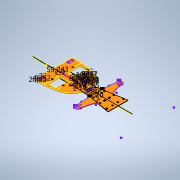
# Autodesk Inventor part: head_1
Saved by Autodesk Inventor 2020 (Build 240168000, 168)
## iProperties
Created: 2022-02-10
Part Number: head_1
Material: Типовые
Document SubType Name: Modeling
Designer: HP
Density: 1 g/cm^3
Appearance: Оранжевый
Mass: 318.083 g
Surface Area: 1630.63 cm^2
Volume: 318.083 cm^3
Author: HP
Autodesk Inventor part; units mm, degrees
ref_plane "YZ Plane" through (0, 0, 0) normal (1, 0, 0) x (0, 1, 0)
ref_plane "XZ Plane" through (0, 0, 0) normal (0, 1, 0) x (-1, 0, 0)
ref_plane "XY Plane" through (0, 0, 0) normal (0, 0, 1) x (1, 0, 0)
sketch "Эскиз1" plane through (0, 0, 0) normal (0, 1, 0) x (-1, 0, 0)
  line L0 (0, 0) -> (-339.521623, 0)
  line L1 (-129.027257, 2.001671) -> (-133.027257, 2.001671) construction
  line L2 (-133.027257, 20.919701) -> (-133.027257, 2.001671) construction
  line L3 (-133.027257, 20.919701) -> (-129.027257, 20.919701) construction
  line L4 (-129.027257, 20.919701) -> (-129.027257, 2.001671) construction
  line L5 (-129.027257, 2.001671) -> (-129.027257, -5.979416)
  line L6 (-10.109935, 0) -> (-40.109935, 0)
  line L7 (-53.743546, -154.136162) -> (-65.871746, -156.19724) construction
  line L8 (-65.871746, -156.19724) -> (-85.372712, -156.989963) construction
  line L9 (-85.372712, -156.989963) -> (-121.679389, -156.038696) construction
  line L10 (-121.679389, -156.038696) -> (-146.412322, -154.136162) construction
  line L11 (-146.412322, -154.136162) -> (-185.097168, -149.221285) construction
  line L12 (-185.097168, -149.221285) -> (-220.928211, -142.879507) construction
  line L13 (-220.928211, -142.879507) -> (-240.429178, -137.64754) construction
  line L14 (-240.429178, -137.64754) -> (-274.35769, -124.963985) construction
  line L15 (-274.35769, -124.963985) -> (-292.748845, -114.024418) construction
  line L16 (-292.748845, -114.024418) -> (-307.334934, -99.596873) construction
  line L17 (-307.334934, -99.596873) -> (-319.384311, -84.53515) construction
  line L18 (-319.384311, -84.53515) -> (-329.372611, -68.205072) construction
  line L19 (-329.372611, -68.205072) -> (-336.665655, -52.667716) construction
  line L20 (-336.665655, -52.667716) -> (-338.102036, -47.843891) construction
  spline S0 degree 4 poles (-53.743546, -154.136162) (-65.871746, -156.19724) (-85.372712, -156.989963) (-121.679389, -156.038696) (-146.412322, -154.136162) (-185.097168, -149.221285) (-220.928211, -142.879507) (-240.429178, -137.64754) (-274.35769, -124.963985) (-292.748845, -114.024418) (-307.334934, -99.596873) (-319.384311, -84.53515) (-329.372611, -68.205072) (-336.665655, -52.667716) (-338.102036, -47.843891) knots 1 1 1 1 1 2 3 4 5 6 7 8 9 10 11 12 12 12 12 12
  line L21 (-338.102036, -47.843891) -> (-338.102036, 0)
  line L22 (-53.743546, 154.136162) -> (-65.871746, 156.19724) construction
  line L23 (-65.871746, 156.19724) -> (-85.372712, 156.989963) construction
  line L24 (-85.372712, 156.989963) -> (-121.679389, 156.038696) construction
  line L25 (-121.679389, 156.038696) -> (-146.412322, 154.136162) construction
  line L26 (-146.412322, 154.136162) -> (-185.097168, 149.221285) construction
  line L27 (-185.097168, 149.221285) -> (-220.928211, 142.879507) construction
  line L28 (-220.928211, 142.879507) -> (-240.429178, 137.64754) construction
  line L29 (-240.429178, 137.64754) -> (-274.35769, 124.963985) construction
  line L30 (-274.35769, 124.963985) -> (-292.748845, 114.024418) construction
  line L31 (-292.748845, 114.024418) -> (-307.334934, 99.596873) construction
  line L32 (-307.334934, 99.596873) -> (-319.384311, 84.53515) construction
  line L33 (-319.384311, 84.53515) -> (-329.372611, 68.205072) construction
  line L34 (-329.372611, 68.205072) -> (-336.665655, 52.667716) construction
  line L35 (-336.665655, 52.667716) -> (-338.102036, 47.843891) construction
  spline S1 degree 4 poles (-53.743546, 154.136162) (-65.871746, 156.19724) (-85.372712, 156.989963) (-121.679389, 156.038696) (-146.412322, 154.136162) (-185.097168, 149.221285) (-220.928211, 142.879507) (-240.429178, 137.64754) (-274.35769, 124.963985) (-292.748845, 114.024418) (-307.334934, 99.596873) (-319.384311, 84.53515) (-329.372611, 68.205072) (-336.665655, 52.667716) (-338.102036, 47.843891) knots 1 1 1 1 1 2 3 4 5 6 7 8 9 10 11 12 12 12 12 12
  line L36 (-338.102036, 47.843891) -> (-338.102036, 0)
  line L37 (-144.743546, 0) -> (-53.743546, 0)
  line L38 (-53.743546, 0) -> (-53.743546, -154.136162)
  line L39 (-53.743546, 154.136162) -> (-65.871746, 156.19724) construction
  line L40 (-65.871746, 156.19724) -> (-85.372712, 156.989963) construction
  line L41 (-85.372712, 156.989963) -> (-121.679389, 156.038696) construction
  line L42 (-121.679389, 156.038696) -> (-146.412322, 154.136162) construction
  line L43 (-146.412322, 154.136162) -> (-185.097168, 149.221285) construction
  line L44 (-185.097168, 149.221285) -> (-220.928211, 142.879507) construction
  line L45 (-220.928211, 142.879507) -> (-240.429178, 137.64754) construction
  line L46 (-240.429178, 137.64754) -> (-274.35769, 124.963985) construction
  line L47 (-274.35769, 124.963985) -> (-292.748845, 114.024418) construction
  line L48 (-292.748845, 114.024418) -> (-307.334934, 99.596873) construction
  line L49 (-307.334934, 99.596873) -> (-319.384311, 84.53515) construction
  line L50 (-319.384311, 84.53515) -> (-329.372611, 68.205072) construction
  line L51 (-329.372611, 68.205072) -> (-336.665655, 52.667716) construction
  line L52 (-336.665655, 52.667716) -> (-338.102036, 47.843891) construction
  spline S2 degree 4 poles (-53.743546, 154.136162) (-65.871746, 156.19724) (-85.372712, 156.989963) (-121.679389, 156.038696) (-146.412322, 154.136162) (-185.097168, 149.221285) (-220.928211, 142.879507) (-240.429178, 137.64754) (-274.35769, 124.963985) (-292.748845, 114.024418) (-307.334934, 99.596873) (-319.384311, 84.53515) (-329.372611, 68.205072) (-336.665655, 52.667716) (-338.102036, 47.843891) knots 1 1 1 1 1 2 3 4 5 6 7 8 9 10 11 12 12 12 12 12
  line L53 (-338.102036, 47.843891) -> (-338.102036, 0)
  line L54 (-53.743546, 0) -> (-53.743546, 154.136162)
  point P0 (-144.743546, 57.777799)
  dimension "d42" = 30
  constraints: 18 end point, 15 symmetric about line, 5 point on line, 2 perpendicular, 1 horizontal, 1 vertical, 9 other
  measures "d42" distance of L6.start L6.end
extrude "Выдавливание1" add sketch "Эскиз1" along normal blind 6
sketch "Эскиз2" plane through (0, 0, 0) normal (0, -1, 0) x (1, 0, 0)
  line L0 (218.921453, 99.86161) -> (218.921453, 139.806254)
  line L1 (218.921453, 139.806254) -> (222.921453, 139.806254)
  line L2 (222.921453, 139.806254) -> (222.921453, 99.86161)
  line L3 (218.921453, 99.86161) -> (222.921453, 99.86161)
  line L4 (218.921453, 59.916966) -> (222.921453, 59.916966)
  line L5 (218.921453, 19.972322) -> (218.921453, 59.916966)
  line L6 (222.921453, 59.916966) -> (222.921453, 19.972322)
  line L7 (218.921453, 19.972322) -> (222.921453, 19.972322)
  line L8 (218.921453, 84.547313) -> (218.921453, 87.447313) construction
  line L9 (222.921453, 87.447313) -> (222.921453, 84.547313) construction
  line L10 (0, 0) -> (287.43499, 0) construction
  line L11 (218.921453, 84.547313) -> (222.921453, 84.547313) construction
  line L12 (222.921453, 84.547313) -> (222.921453, 87.447313) construction
  line L13 (222.921453, 87.447313) -> (218.921453, 87.447313) construction
  line L14 (218.921453, 87.447313) -> (218.921453, 84.547313) construction
  line L15 (218.921453, 84.547313) -> (222.921453, 87.447313) construction
  line L16 (222.921453, 84.547313) -> (218.921453, 87.447313) construction
  circle A0 centre (220.921453, 85.997313) radius 1.5
  line L17 (218.921453, -99.86161) -> (218.921453, -139.806254)
  line L18 (218.921453, -139.806254) -> (222.921453, -139.806254)
  line L19 (222.921453, -139.806254) -> (222.921453, -99.86161)
  line L20 (218.921453, -99.86161) -> (222.921453, -99.86161)
  line L21 (218.921453, -59.916966) -> (222.921453, -59.916966)
  line L22 (218.921453, -19.972322) -> (218.921453, -59.916966)
  line L23 (222.921453, -59.916966) -> (222.921453, -19.972322)
  line L24 (218.921453, -19.972322) -> (222.921453, -19.972322)
  line L25 (218.921453, -84.547313) -> (218.921453, -87.447313) construction
  line L26 (222.921453, -87.447313) -> (222.921453, -84.547313) construction
  line L27 (218.921453, -84.547313) -> (222.921453, -84.547313) construction
  line L28 (222.921453, -84.547313) -> (222.921453, -87.447313) construction
  line L29 (222.921453, -87.447313) -> (218.921453, -87.447313) construction
  line L30 (218.921453, -87.447313) -> (218.921453, -84.547313) construction
  line L31 (218.921453, -84.547313) -> (222.921453, -87.447313) construction
  line L32 (222.921453, -84.547313) -> (218.921453, -87.447313) construction
  circle A1 centre (220.921453, -85.997313) radius 1.5
  dimension "d101" = 3
  constraints: 66 end point, 16 symmetric about line, 6 horizontal, 6 vertical, 4 midpoint, 2 centre point, 2 coincident, 2 parallel, 1 perpendicular, 13 other
  measures "d101" diameter of A0
sketch "Эскиз6" plane through (0, 0, 0) normal (0, -1, 0) x (1, 0, 0)
  line L0 (74.395998, 0) -> (255.779052, 0)
  line L1 (174.802002, 33.285159) -> (169.607709, 33.285159)
  line L2 (180.665084, 129.150848) -> (169.607709, 129.150848)
  line L3 (145.357709, 104.101025) -> (145.357709, 81.101025)
  line L4 (142.506422, 31.26111) -> (204.162039, 31.26111)
  line L5 (204.162039, 31.26111) -> (204.162039, 131.44265)
  line L6 (204.162039, 131.44265) -> (142.506422, 131.44265)
  line L7 (142.506422, 131.44265) -> (142.506422, 31.26111)
  line L8 (174.802002, -33.285159) -> (169.607709, -33.285159)
  line L9 (180.665084, -129.150848) -> (169.607709, -129.150848)
  line L10 (145.357709, -104.101025) -> (145.357709, -81.101025)
  line L11 (142.506422, -31.26111) -> (204.162039, -31.26111)
  line L12 (204.162039, -31.26111) -> (204.162039, -131.44265)
  line L13 (204.162039, -131.44265) -> (142.506422, -131.44265)
  line L14 (142.506422, -131.44265) -> (142.506422, -31.26111)
  point P0 (0, 0)
  constraints: 24 end point, 10 symmetric about line, 2 horizontal, 2 parallel, 1 perpendicular
sketch "Эскиз7" plane through (0, 0, 0) normal (0, -1, 0) x (1, 0, 0)
  point P0 (0, 0)
extrude "Выдавливание10" cut sketch "Эскиз6" against normal through all
sketch "Эскиз11" plane through (0, 6, 0) normal (0, 1, 0) x (1, 0, 0)
  line L0 (53.743546, 154.136162) -> (53.743546, -154.136162)
  line L1 (338.102036, -47.843891) -> (338.102036, 47.843891)
  point P0 (0, 0)
  constraints: 2 other
sketch "Эскиз12" plane through (0, 0, 0) normal (0, -1, 0) x (1, 0, 0)
  line L0 (232.5, 139.475161) -> (232.5, 54.475161)
  circle A0 centre (232.5, 54.475161) radius 0.05
  point P0 (0, 0)
  dimension "d56" = 85
  dimension "d60" = 0.1
  constraints: 2 coincident, 2 end point, 1 centre point, 1 vertical, 2 other
  measures "d56" distance of L0.start L0.end
  measures "d60" diameter of A0
extrude "Выдавливание12" cut sketch "Эскиз12" against normal blind 0.1
sketch "Эскиз13" plane through (0, 6, 0) normal (0, 1, 0) x (1, 0, 0)
  point P0 (0, 0)
  point P1 (303.305898, -69.722631)
sketch "Эскиз18" plane through (0, 0, 0) normal (0, -1, 0) x (1, 0, 0)
  line L0 (127.94871, -106.917014) -> (127.94871, -149.683819)
  line L1 (131.94871, -149.683819) -> (131.94871, -106.917014)
  line L2 (127.94871, -149.683819) -> (131.94871, -149.683819)
  line L3 (131.94871, -106.917014) -> (127.94871, -106.917014)
  line L4 (127.94871, -64.150208) -> (131.94871, -64.150208)
  line L5 (127.94871, -21.383403) -> (127.94871, -64.150208)
  line L6 (131.94871, -64.150208) -> (131.94871, -21.383403)
  line L7 (131.94871, -21.383403) -> (127.94871, -21.383403)
  line L8 (127.94871, -86.983611) -> (127.94871, -84.083611) construction
  line L9 (131.94871, -84.083611) -> (131.94871, -86.983611) construction
  line L10 (127.94871, -86.983611) -> (131.94871, -86.983611) construction
  line L11 (131.94871, -86.983611) -> (131.94871, -84.083611) construction
  line L12 (131.94871, -84.083611) -> (127.94871, -84.083611) construction
  line L13 (127.94871, -84.083611) -> (127.94871, -86.983611) construction
  line L14 (127.94871, -86.983611) -> (131.94871, -84.083611) construction
  line L15 (131.94871, -86.983611) -> (127.94871, -84.083611) construction
  circle A0 centre (129.94871, -85.533611) radius 1.5
  line L16 (0, 0) -> (309.38051, 0) construction
  line L17 (127.94871, 106.917014) -> (127.94871, 149.683819)
  line L18 (131.94871, 149.683819) -> (131.94871, 106.917014)
  line L19 (127.94871, 149.683819) -> (131.94871, 149.683819)
  line L20 (131.94871, 106.917014) -> (127.94871, 106.917014)
  line L21 (127.94871, 64.150208) -> (131.94871, 64.150208)
  line L22 (127.94871, 21.383403) -> (127.94871, 64.150208)
  line L23 (131.94871, 64.150208) -> (131.94871, 21.383403)
  line L24 (131.94871, 21.383403) -> (127.94871, 21.383403)
  line L25 (127.94871, 86.983611) -> (127.94871, 84.083611) construction
  line L26 (131.94871, 84.083611) -> (131.94871, 86.983611) construction
  line L27 (127.94871, 86.983611) -> (131.94871, 86.983611) construction
  line L28 (131.94871, 86.983611) -> (131.94871, 84.083611) construction
  line L29 (131.94871, 84.083611) -> (127.94871, 84.083611) construction
  line L30 (127.94871, 84.083611) -> (127.94871, 86.983611) construction
  line L31 (127.94871, 86.983611) -> (131.94871, 84.083611) construction
  line L32 (131.94871, 86.983611) -> (127.94871, 84.083611) construction
  circle A1 centre (129.94871, 85.533611) radius 1.5
  dimension "d96" = 3
  constraints: 66 end point, 16 symmetric about line, 6 horizontal, 6 vertical, 4 midpoint, 2 centre point, 2 coincident, 2 parallel, 1 perpendicular, 13 other
  measures "d96" diameter of A0
extrude "Выдавливание22" cut sketch "Эскиз18" against normal blind 10
extrude "Выдавливание23" cut sketch "Эскиз2" against normal through all
sketch "Эскиз19" plane through (0, 6, 0) normal (0, 1, 0) x (1, 0, 0)
  line L0 (590.53404, -82.183099) -> (370.53404, -45)
  line L1 (590.53404, 82.183099) -> (590.53404, -82.183099) construction
  line L2 (370.53404, -45) -> (204.162039, -45)
  line L3 (590.53404, 0) -> (590.53404, -82.183099)
  line L4 (222.921453, 139.806254) -> (222.921453, 99.86161)
  line L5 (222.921453, 99.86161) -> (218.921453, 99.86161)
  line L6 (218.921453, 99.86161) -> (218.921453, 139.806254)
  line L7 (218.921453, 139.806254) -> (222.921453, 139.806254)
  circle A0 centre (220.921453, -85.997313) radius 1.5
  line L8 (222.921453, -139.806254) -> (218.921453, -139.806254)
  line L9 (218.921453, -139.806254) -> (218.921453, -99.86161)
  line L10 (218.921453, -99.86161) -> (222.921453, -99.86161)
  line L11 (222.921453, -99.86161) -> (222.921453, -139.806254)
  line L12 (222.921453, 19.972322) -> (218.921453, 19.972322)
  line L13 (218.921453, 19.972322) -> (218.921453, 59.916966)
  line L14 (218.921453, 59.916966) -> (222.921453, 59.916966)
  line L15 (222.921453, 59.916966) -> (222.921453, 19.972322)
  circle A1 centre (220.921453, 85.997313) radius 1.5
  line L16 (218.921453, -19.972322) -> (222.921453, -19.972322)
  line L17 (222.921453, -19.972322) -> (222.921453, -59.916966)
  line L18 (222.921453, -59.916966) -> (218.921453, -59.916966)
  line L19 (218.921453, -59.916966) -> (218.921453, -19.972322)
  line L20 (127.94871, 106.917014) -> (127.94871, 149.683819)
  line L21 (127.94871, 149.683819) -> (131.94871, 149.683819)
  line L22 (131.94871, 149.683819) -> (131.94871, 106.917014)
  line L23 (131.94871, 106.917014) -> (127.94871, 106.917014)
  line L24 (127.94871, -21.383403) -> (131.94871, -21.383403)
  line L25 (131.94871, -21.383403) -> (131.94871, -64.150208)
  line L26 (131.94871, -64.150208) -> (127.94871, -64.150208)
  line L27 (127.94871, -64.150208) -> (127.94871, -21.383403)
  line L28 (127.94871, 21.383403) -> (127.94871, 64.150208)
  line L29 (127.94871, 64.150208) -> (131.94871, 64.150208)
  line L30 (131.94871, 64.150208) -> (131.94871, 21.383403)
  line L31 (131.94871, 21.383403) -> (127.94871, 21.383403)
  circle A2 centre (129.94871, 85.533611) radius 1.5
  circle A3 centre (129.94871, -85.533611) radius 1.5
  line L32 (127.94871, -149.683819) -> (127.94871, -106.917014)
  line L33 (127.94871, -106.917014) -> (131.94871, -106.917014)
  line L34 (131.94871, -106.917014) -> (131.94871, -149.683819)
  line L35 (131.94871, -149.683819) -> (127.94871, -149.683819)
  line L36 (132.908073, -2) -> (132.908073, 2)
  line L37 (132.908073, 2) -> (192.597533, 2)
  line L38 (192.597533, 2) -> (192.597533, -2)
  line L39 (192.597533, -2) -> (132.908073, -2)
  circle A4 centre (252.499965, -54.504877) radius 1.5
  circle A5 centre (252.489072, -26.566338) radius 1.5
  circle A6 centre (304.82708, -21.46988) radius 1.5
  line L40 (204.162039, -31.26111) -> (204.162039, -131.44265)
  line L41 (204.162039, -131.44265) -> (142.506422, -131.44265)
  line L42 (142.506422, -131.44265) -> (142.506422, -31.26111)
  line L43 (142.506422, -31.26111) -> (204.162039, -31.26111)
  line L44 (204.162039, 31.26111) -> (142.506422, 31.26111)
  line L45 (142.506422, 31.26111) -> (142.506422, 131.44265)
  line L46 (142.506422, 131.44265) -> (204.162039, 131.44265)
  line L47 (204.162039, 131.44265) -> (204.162039, 31.26111)
  line L48 (338.102036, -47.843891) -> (338.102036, 47.843891)
  spline S0 degree 4 poles (338.102036, 47.843891) (336.665655, 52.667716) (329.372611, 68.205072) (319.384311, 84.53515) (307.334934, 99.596873) (292.748845, 114.024418) (274.35769, 124.963985) (240.429178, 137.64754) (220.928211, 142.879507) (185.097168, 149.221285) (146.412322, 154.136162) (121.679389, 156.038696) (85.372712, 156.989963) (65.871746, 156.19724) (53.743546, 154.136162) knots 1 1 1 1 1 2 3 4 5 6 7 8 9 10 11 12 12 12 12 12
  line L49 (53.743546, 154.136162) -> (53.743546, -154.136162)
  spline S1 degree 4 poles (53.743546, -154.136162) (65.871746, -156.19724) (85.372712, -156.989963) (121.679389, -156.038696) (146.412322, -154.136162) (185.097168, -149.221285) (220.928211, -142.879507) (240.429178, -137.64754) (274.35769, -124.963985) (292.748845, -114.024418) (307.334934, -99.596873) (319.384311, -84.53515) (329.372611, -68.205072) (336.665655, -52.667716) (338.102036, -47.843891) knots 1 1 1 1 1 2 3 4 5 6 7 8 9 10 11 12 12 12 12 12
  circle A7 centre (366.494375, -34.175417) radius 1.5
  circle A8 centre (433.543463, -45.507657) radius 1.5
  circle A9 centre (433.543463, -22.843176) radius 1.5
  circle A10 centre (500.592552, -56.839897) radius 1.5
  circle A11 centre (500.592552, -22.843176) radius 1.5
  circle A12 centre (500.592552, -14.75) radius 1.45
  circle A13 centre (567.641641, -68.172138) radius 1.5
  circle A14 centre (567.641641, -22.843176) radius 1.5
  circle A15 centre (366.494375, 0) radius 1.5
  line L50 (590.53404, 0) -> (556.709794, 0)
  line L51 (590.53404, 0) -> (557.964133, 0)
  line L52 (590.53404, 82.183099) -> (370.53404, 45)
  line L53 (590.53404, 0) -> (590.53404, 82.183099)
  circle A16 centre (366.494375, 34.175417) radius 1.5
  circle A17 centre (433.543463, 45.507657) radius 1.5
  circle A18 centre (433.543463, 22.843176) radius 1.5
  circle A19 centre (500.592552, 56.839897) radius 1.5
  circle A20 centre (500.592552, 22.843176) radius 1.5
  circle A21 centre (500.592552, 14.75) radius 1.45
  circle A22 centre (567.641641, 68.172138) radius 1.5
  circle A23 centre (567.641641, 22.843176) radius 1.5
  circle A24 centre (366.494375, 0) radius 1.5
  line L54 (370.53404, 45) -> (204.162039, 45)
  line L55 (204.162039, -31.26111) -> (204.162039, -131.44265)
  line L56 (204.162039, 131.44265) -> (204.162039, 31.26111)
  circle A25 centre (348.506066, -17.087708) radius 8
  circle A26 centre (304.839956, -21.484903) radius 1.5
  circle A27 centre (303.29996, -69.744885) radius 1.5
  circle A28 centre (252.499965, -26.564858) radius 1.5
  circle A29 centre (252.499965, -54.504877) radius 1.5
  line L57 (366.494375, -34.175417) -> (366.494375, 0)
  line L58 (-118.106808, 0) -> (708.640848, 0)
  circle A30 centre (348.506066, 17.087708) radius 8
  circle A31 centre (348.506066, -17.087708) radius 9.5
  circle A32 centre (348.506066, 17.087708) radius 9.5
  line L59 (366.494375, -34.175417) -> (434.494375, -34.175417) construction
  circle A33 centre (299.444666, -22.846844) radius 1.5
  line L60 (299.444666, -22.846844) -> (367.444666, -22.846844) construction
  circle A34 centre (232.394957, -11.518271) radius 1.5
  circle A35 centre (299.444666, 22.846844) radius 1.5
  circle A36 centre (232.394957, 11.518271) radius 1.5
  point P0 (0, 0)
  point P1 (338.102036, 45)
  point P2 (338.102036, -45)
  point P3 (305.972405, -20.501257)
  point P4 (303.694631, -22.453526)
  point P5 (252.292545, -25.079268)
  point P6 (252.696492, -28.051928)
  point P7 (366.494375, -17.087708)
  dimension "d118" = 16
  dimension "d190" = 19
  dimension "d215" = 3
  constraints: 37 centre point, 24 end point, 12 symmetric about line, 5 equal radius, 5 horizontal, 3 vertical, 2 coincident, 2 midpoint, 1 point on line, 39 other
  measures "d118" diameter of A25
  measures "d190" diameter of A31
  measures "d215" diameter of A33
sketch "Эскиз20" plane through (0, 6, 0) normal (0, 1, 0) x (1, 0, 0)
  line L0 (338.102036, -47.843891) -> (338.102036, 47.843891)
  line L1 (370.53404, -45) -> (150.53404, -45)
  line L2 (338.102036, -45) -> (398.310009, -45) construction
  circle A0 centre (313.494375, 0) radius 1.5
  circle A1 centre (313.494375, 0) radius 1.5
  line L3 (313.494375, 0) -> (378.494375, 0)
  circle A2 centre (378.494375, 0) radius 2.5
  line L4 (378.494375, 0) -> (408.494375, 0)
  line L5 (590.53404, -82.183099) -> (496.225076, -66.243556)
  line L6 (370.53404, 45) -> (590.53404, 82.183099)
  line L7 (150.53404, 45) -> (370.53404, 45)
  line L8 (408.494375, 0) -> (408.494375, -51.415831)
  line L9 (408.494375, 51.415831) -> (408.494375, 0)
  spline S0 degree 2 poles (408.494375, -51.415831) (407.497612, -115.458679) (417.984162, -180.733061) knots 0 0 0 1 1 1
  arc A3 (417.984162, -180.733061) -> (450.061396, -183.259047) centre (434.721088, -173.128293) ccw
  spline S1 degree 2 poles (408.494375, 51.415831) (407.497612, 115.458679) (417.984162, 180.733061) knots 0 0 0 1 1 1
  arc A4 (450.061396, 183.259047) -> (417.984162, 180.733061) centre (434.721088, 173.128293) ccw
  line L10 (590.53404, -82.183099) -> (370.53404, -45)
  line L11 (338.102036, -47.843891) -> (338.102036, 47.843891)
  line L12 (313.494375, 0) -> (338.102036, 0)
  line L13 (708.640848, 0) -> (-118.106808, 0)
  line L14 (53.743546, 154.136162) -> (53.743546, -154.136162)
  line L15 (53.743546, 0) -> (112.615546, 0)
  line L16 (53.743546, 0) -> (112.986546, 0)
  line L17 (112.986546, 0) -> (110.086546, 0)
  circle A5 centre (111.536546, 0) radius 1.45
  line L18 (460.711317, -60.24123) -> (480.431637, -63.574242)
  arc A6 (474.217889, -78.803208) -> (450.061396, -183.259047) centre (835.740939, -217.43029) ccw
  arc A7 (496.225076, -66.243556) -> (474.217889, -78.803208) centre (492.892065, -85.963876) ccw
  arc A8 (450.061396, 183.259047) -> (417.984162, 180.733061) centre (434.721088, 173.128293) ccw
  arc A9 (450.061396, 183.259047) -> (474.217889, 78.803208) centre (835.740939, 217.43029) ccw
  arc A10 (474.217889, 78.803208) -> (496.225076, 66.243556) centre (492.892065, 85.963876) ccw
  point P0 (0, 0)
  point P1 (453.008626, -171.251285)
  point P2 (432.734599, -153.77409)
  point P3 (453.008626, 171.251285)
  point P4 (432.734599, 153.77409)
  point P5 (450.863733, 150.353763)
  dimension "d106" = 65
  dimension "d107" = 5
  dimension "d110" = 30
  dimension "d225" = 3
  dimension "d240" = 59.243
  dimension "d241" = 2.9
  dimension "d260" = 20
  constraints: 30 end point, 15 point on circle, 10 centre point, 9 point on line, 6 vertical alignment, 5 symmetric about line, 4 horizontal, 3 equal radius, 3 midpoint, 2 coincident, 2 tangent, 1 collinear, 1 horizontal alignment, 1 perpendicular, 1 vertical, 28 other
  measures "d106" distance of L3.start L3.end
  measures "d107" diameter of A2
  measures "d110" distance of L4.start L4.end
  measures "d225" diameter of A0
  measures "d240" distance of L15.start L16.end
  measures "d241" distance of L16.end L17.end
  measures "d260" radius of A7
extrude "Выдавливание24" add sketch "Эскиз19" against normal blind 6 contours L0 L2 L48 L58 A15 L50 L3 | L50 L58 A15 L48 L54 L52 L53 | A25 | A30 | A31 | A32
extrude "Выдавливание25" add sketch "Эскиз20" against normal blind 6 contours L10 A7 A6 A3 S0
sketch "Эскиз34" plane through (0, 0, 0) normal (0, -1, 0) x (1, 0, 0)
  line L0 (147.451162, 2) -> (147.451162, -2)
  line L1 (147.451162, -2) -> (194.844244, -2)
  line L2 (194.844244, 2) -> (147.451162, 2)
  line L3 (194.844244, -2) -> (194.844244, 2)
  line L4 (242.237326, 2) -> (242.237326, -2)
  line L5 (242.237326, -2) -> (289.630407, -2)
  line L6 (289.630407, 2) -> (242.237326, 2)
  line L7 (289.630407, -2) -> (289.630407, 2)
  line L8 (52.664999, -2) -> (100.058081, -2)
  line L9 (100.058081, 2) -> (52.664999, 2)
  line L10 (100.058081, -2) -> (100.058081, 2)
  line L11 (52.664999, 2) -> (52.664999, -2)
  point P0 (0, 0)
  constraints: 24 end point, 6 horizontal, 6 vertical, 12 other
extrude "Выдавливание43" cut sketch "Эскиз34" against normal blind 6
extrude "Выдавливание26" cut sketch "Эскиз20" against normal blind 6 contours A2 L4 L3 | L3 L4 A2 | L3 L13 A0 | A0 L13 L3
extrude "Выдавливание27" cut sketch "Эскиз19" against normal blind 6 contours A25
sketch "Эскиз21" plane through (0, 6, 0) normal (0, 1, 0) x (1, 0, 0)
  point P0 (0, 0)
sketch "Эскиз22" plane through (0, 6, 0) normal (0, 1, 0) x (1, 0, 0)
  line L0 (272.616718, 69.365757) -> (272.616718, 26.185757)
  line L1 (272.616718, 26.185757) -> (293.698718, 26.185757)
  line L2 (293.698718, 26.185757) -> (293.698718, 69.365757)
  line L3 (293.698718, 69.365757) -> (272.616718, 69.365757)
  line L4 (293.698718, 69.365757) -> (293.698718, 62.761757)
  line L5 (283.157718, 69.365757) -> (291.730218, 69.365757)
  circle A0 centre (291.730218, 62.761757) radius 1.44
  line L6 (272.616718, 26.185757) -> (272.616718, 32.789757)
  circle A1 centre (274.585303, 33.099696) radius 1.44
  line L7 (293.698718, 62.761757) -> (293.170218, 62.761757)
  line L8 (246.593604, 26.185757) -> (246.593604, 69.365757)
  line L9 (246.593604, 69.365757) -> (225.511604, 69.365757)
  line L10 (225.511604, 69.365757) -> (225.511604, 26.185757)
  line L11 (225.511604, 26.185757) -> (246.593604, 26.185757)
  line L12 (294.698803, 68.675696) -> (294.698803, 62.071696)
  line L13 (236.052604, 26.185757) -> (227.480104, 26.185757)
  circle A2 centre (227.480104, 32.789757) radius 1.44
  circle A3 centre (244.625104, 62.761757) radius 1.44
  line L14 (294.698803, 62.071696) -> (294.170303, 62.071696)
  circle A4 centre (251.765737, 32.789757) radius 1.44
  line L15 (249.816991, 26.185757) -> (270.898991, 26.185757)
  line L16 (249.816991, 69.365757) -> (249.816991, 26.185757)
  line L17 (270.898991, 26.185757) -> (270.898991, 69.365757)
  circle A5 centre (268.680505, 62.761757) radius 1.44
  line L18 (270.898991, 69.365757) -> (249.816991, 69.365757)
  line L19 (227.480104, 26.185757) -> (227.480104, 32.789757)
  line L20 (227.480104, 32.789757) -> (225.511604, 32.789757)
  line L21 (268.680505, 62.761757) -> (268.680505, 69.365757)
  line L22 (244.625104, 62.761757) -> (244.625104, 69.365757)
  line L23 (251.765737, 32.789757) -> (251.765737, 26.185757)
  line L24 (246.593604, 69.365757) -> (244.625104, 69.365757)
  point P0 (0, 0)
  point P1 (294.170303, 62.071696)
  point P2 (295.170303, 61.071696)
  dimension "d125" = 2.88
  dimension "d121" = 43.18
  dimension "d122" = 21.082
  dimension "d123" = 6.604
  dimension "d124" = 8.5725
  dimension "d126" = 6.604
  dimension "d128" = 2.88
  dimension "d129" = 0.5285
  dimension "d156" = 21.082
  dimension "d157" = 6.604
  dimension "d158" = 8.5725
  dimension "d159" = 2.88
  dimension "d163" = 0.5285
  dimension "d171" = 43.18
  dimension "d175" = 6.604
  dimension "d176" = 1.9685
  constraints: 50 end point, 11 parallel, 8 point on line, 6 perpendicular, 5 centre point, 3 equal radius, 2 collinear, 2 midpoint, 1 horizontal alignment, 2 other
  measures "d121" distance of L2.end L1.end
  measures "d122" distance of L1.end L0.end
  measures "d123" distance of L2.end L4.end
  measures "d124" distance of L5.start L5.end
  measures "d126" distance of L0.end L6.end
  measures "d128" diameter of A1
  measures "d129" distance of L4.end L7.end
  measures "d156" distance of L9.end L9.start
  measures "d157" distance of L12.start L14.start
  measures "d158" distance of L13.start L13.end
  measures "d159" diameter of A2
  measures "d163" distance of L14.start L14.end
  measures "d171" distance of L8.start L9.start
  measures "d175" distance of L22.start L22.end
  measures "d176" distance of L9.start L22.end
extrude "Выдавливание28" cut sketch "Эскиз22" against normal blind 6 contours A0 | A1
sketch "Эскиз19 outline for Выдавливание29" plane through (0, 6, 0) normal (0, 1, 0) x (1, 0, 0)
  arc A0 (305.972405, -20.501257) -> (303.694631, -22.453526) centre (304.839956, -21.484903) ccw
  arc A1 (303.694631, -22.453526) -> (305.972405, -20.501257) centre (304.82708, -21.46988) ccw
  arc A2 (252.292545, -25.079268) -> (252.696492, -28.051928) centre (252.499965, -26.564858) ccw
  arc A3 (252.696492, -28.051928) -> (252.292545, -25.079268) centre (252.489072, -26.566338) ccw
  circle A4 centre (303.29996, -69.744885) radius 1.5
  circle A5 centre (252.499965, -54.504877) radius 1.5
extrude "Выдавливание29" cut sketch "Эскиз19 outline for Выдавливание29" against normal blind 6
sketch "Эскиз24" plane through (0, 6, 0) normal (0, 1, 0) x (1, 0, 0)
  circle A0 centre (252.499965, -54.504877) radius 1.5
  circle A1 centre (252.489072, -26.566338) radius 1.5
  circle A2 centre (304.82708, -21.46988) radius 1.5
  circle A3 centre (304.839956, -21.484903) radius 1.5
  circle A4 centre (303.29996, -69.744885) radius 1.5
  circle A5 centre (252.499965, -26.564858) radius 1.5
  circle A6 centre (252.499965, -54.504877) radius 1.5
  circle A7 centre (252.499965, -54.504877) radius 1.5
  circle A8 centre (252.489072, -26.566338) radius 1.5
  circle A9 centre (304.82708, -21.46988) radius 1.5
  circle A10 centre (304.839956, -21.484903) radius 1.5
  circle A11 centre (303.29996, -69.744885) radius 1.5
  circle A12 centre (252.499965, -26.564858) radius 1.5
  circle A13 centre (252.499965, -54.504877) radius 1.5
  point P0 (0, 0)
  dimension "d141" = 3
  dimension "d142" = 3
  constraints: 20 centre point, 6 equal radius
  measures "d141" diameter of A3
  measures "d142" diameter of A10
sketch "Эскиз25" plane through (0, 6, 0) normal (0, 1, 0) x (1, 0, 0)
  circle A0 centre (81.981142, 102.339991) radius 1.5
  circle A1 centre (109.91968, 102.350884) radius 1.5
  circle A2 centre (115.016139, 50.012877) radius 1.5
  circle A3 centre (115.001115, 50) radius 1.5
  circle A4 centre (66.50538, 51.540412) radius 1.5
  circle A5 centre (109.92116, 102.339991) radius 1.5
  circle A6 centre (81.981142, 102.339991) radius 1.5
  line L0 (-118.106808, 0) -> (708.640848, 0)
  circle A7 centre (99.304624, -100.798453) radius 1.5
  circle A8 centre (115.001115, -50) radius 1.5
  circle A9 centre (66.50538, -48.471755) radius 1.5
  circle A10 centre (71.364605, -100.798453) radius 1.5
  line L1 (132.908073, -2) -> (132.908073, 2)
  line L2 (69.825662, -13.240842) -> (71.825662, -13.240842)
  line L3 (71.825662, -13.240842) -> (71.825662, -9.240842)
  line L4 (71.825662, -9.240842) -> (69.825662, -9.240842)
  line L5 (69.825662, -9.240842) -> (69.825662, -13.240842)
  line L6 (86.825662, -13.240842) -> (88.825662, -13.240842)
  line L7 (88.825662, -13.240842) -> (88.825662, -9.240842)
  line L8 (88.825662, -9.240842) -> (86.825662, -9.240842)
  line L9 (86.825662, -9.240842) -> (86.825662, -13.240842)
  line L10 (69.825662, 13.240842) -> (71.825662, 13.240842)
  line L11 (71.825662, 13.240842) -> (71.825662, 9.240842)
  line L12 (71.825662, 9.240842) -> (69.825662, 9.240842)
  line L13 (69.825662, 9.240842) -> (69.825662, 13.240842)
  line L14 (86.825662, 13.240842) -> (88.825662, 13.240842)
  line L15 (88.825662, 13.240842) -> (88.825662, 9.240842)
  line L16 (88.825662, 9.240842) -> (86.825662, 9.240842)
  line L17 (86.825662, 9.240842) -> (86.825662, 13.240842)
  line L18 (251.413455, 11.187786) -> (253.413455, 11.187786)
  line L19 (253.413455, 11.187786) -> (253.413455, 15.187786)
  line L20 (253.413455, 15.187786) -> (251.413455, 15.187786)
  line L21 (251.413455, 15.187786) -> (251.413455, 11.187786)
  line L22 (268.413455, 11.187786) -> (270.413455, 11.187786)
  line L23 (270.413455, 11.187786) -> (270.413455, 15.187786)
  line L24 (270.413455, 15.187786) -> (268.413455, 15.187786)
  line L25 (268.413455, 15.187786) -> (268.413455, 11.187786)
  line L26 (117.431454, 26.92188) -> (97.431454, 26.92188)
  line L27 (97.431454, 26.92188) -> (97.431454, 6.92188)
  line L28 (97.431454, 6.92188) -> (117.431454, 6.92188)
  line L29 (117.431454, 6.92188) -> (117.431454, 26.92188)
  line L30 (97.431454, 16.92188) -> (99.435231, 16.92188)
  line L31 (99.435231, 16.92188) -> (99.435231, 7.62188)
  line L32 (99.435231, 7.62188) -> (99.435231, 26.22188)
  circle A11 centre (99.435231, 7.62188) radius 0.5
  circle A12 centre (99.435231, 26.22188) radius 0.5
  line L33 (117.431454, -26.92188) -> (97.431454, -26.92188)
  line L34 (97.431454, -26.92188) -> (97.431454, -6.92188)
  line L35 (97.431454, -6.92188) -> (117.431454, -6.92188)
  line L36 (117.431454, -6.92188) -> (117.431454, -26.92188)
  line L37 (97.431454, -16.92188) -> (99.435231, -16.92188)
  line L38 (99.435231, -16.92188) -> (99.435231, -7.62188)
  line L39 (99.435231, -7.62188) -> (99.435231, -26.22188)
  circle A13 centre (99.435231, -7.62188) radius 0.5
  circle A14 centre (99.435231, -26.22188) radius 0.5
  point P0 (0, 0)
  point P1 (111.40675, 102.547411)
  point P2 (108.43409, 102.143464)
  dimension "d143" = 3
  dimension "d208" = 4
  dimension "d209" = 2
  dimension "d210" = 15
  dimension "d244" = 4
  dimension "d245" = 2
  dimension "d246" = 15
  dimension "d249" = 20
  dimension "d250" = 20
  dimension "d251" = 9.3
  dimension "d252" = 18.6
  dimension "d253" = 1
  dimension "d254" = 1
  constraints: 76 end point, 20 centre point, 18 symmetric about line, 10 parallel, 6 horizontal, 6 perpendicular, 4 coincident, 4 equal length, 3 equal radius, 2 collinear, 2 point on line, 1 midpoint, 2 other
  measures "d143" diameter of A3
  measures "d208" distance of L4.end L2.start
  measures "d209" distance of L3.end L4.end
  measures "d210" distance between parallel lines of L9 L3
  measures "d244" distance of L20.end L18.start
  measures "d245" distance of L20.start L20.end
  measures "d246" distance between parallel lines of L25 L19
  measures "d249" distance of L28.end L27.end
  measures "d250" distance of L27.end L26.end
  measures "d251" distance of L30.end L31.end
  measures "d252" distance of L31.end L32.end
  measures "d253" diameter of A11
  measures "d254" diameter of A12
sketch "Эскиз25 outline for Выдавливание30" plane through (0, 6, 0) normal (0, 1, 0) x (1, 0, 0)
  arc A0 (111.40675, 102.547411) -> (108.43409, 102.143464) centre (109.92116, 102.339991) ccw
  arc A1 (108.43409, 102.143464) -> (111.40675, 102.547411) centre (109.91968, 102.350884) ccw
  circle A2 centre (81.981142, 102.339991) radius 1.5
  circle A3 centre (66.50538, 51.540412) radius 1.5
  circle A4 centre (115.001115, 50) radius 1.5
extrude "Выдавливание30" cut sketch "Эскиз25 outline for Выдавливание30" against normal blind 6
sketch "Эскиз27" plane through (0, 6, 0) normal (0, 1, 0) x (1, 0, 0)
  circle A0 centre (236.226018, 115.676477) radius 1.5
  circle A1 centre (236.226018, 89.776477) radius 1.5
  line L0 (236.226018, 89.776477) -> (236.226018, 115.676477)
  line L1 (236.226018, 115.676477) -> (236.226018, 123.845404)
  line L2 (82.944066, -98.472535) -> (82.944066, -144.992535)
  line L3 (82.944066, -144.992535) -> (62.694066, -144.992535)
  line L4 (62.694066, -144.992535) -> (62.694066, -98.472535)
  line L5 (62.694066, -98.472535) -> (82.944066, -98.472535)
  line L6 (246.351018, 125.986477) -> (229.83238, 69.513191) construction
  line L7 (250.08238, 69.513191) -> (226.101018, 125.986477) construction
  circle A2 centre (72.819203, -108.0173) radius 1.5
  circle A3 centre (72.819203, -133.9173) radius 1.5
  line L8 (247.351018, 126.986477) -> (247.351018, 80.466477)
  line L9 (247.351018, 80.466477) -> (227.101018, 80.466477)
  line L10 (227.101018, 80.466477) -> (227.101018, 126.986477)
  line L11 (227.101018, 126.986477) -> (247.351018, 126.986477)
  line L12 (708.640848, 0) -> (-118.106808, 0)
  line L13 (708.640848, 0) -> (-118.106808, 0)
  line L14 (0, 0) -> (20.000346, 0)
  line L15 (82.944066, 98.472535) -> (82.944066, 144.992535)
  line L16 (82.944066, 144.992535) -> (62.694066, 144.992535)
  line L17 (62.694066, 144.992535) -> (62.694066, 98.472535)
  line L18 (62.694066, 98.472535) -> (82.944066, 98.472535)
  circle A4 centre (72.819203, 133.9173) radius 1.5
  circle A5 centre (72.819203, 108.0173) radius 1.5
  point P0 (236.226018, 102.726477)
  dimension "d146" = 3
  dimension "d147" = 3
  dimension "d148" = 25.9
  dimension "d177" = 46.52
  dimension "d178" = 20.25
  dimension "d229" = 3
  dimension "d230" = 3
  dimension "d232" = 46.52
  dimension "d233" = 20.25
  constraints: 38 end point, 6 centre point, 6 symmetric about line, 4 parallel, 2 horizontal, 2 perpendicular, 2 vertical, 1 midpoint, 1 point on line, 6 other
  measures "d146" diameter of A0
  measures "d147" diameter of A1
  measures "d148" distance of L0.start L0.end
  measures "d177" distance of L2.start L2.end
  measures "d178" distance of L2.end L3.end
  measures "d229" diameter of A2
  measures "d230" diameter of A3
  measures "d232" distance of L11.end L9.start
  measures "d233" distance of L9.start L10.start
extrude "Выдавливание31" cut sketch "Эскиз27" against normal blind 6 contours A0 L0 L1 | L1 L0 A0 | A1
extrude "Выдавливание32" cut sketch "Эскиз22" against normal blind 6 contours L19 L20 A2 | A2 L20 L19 | A3 | A4 | A5
sketch "Эскиз28" plane through (0, 6, 0) normal (0, 1, 0) x (1, 0, 0)
  line L0 (378.497279, 0) -> (358.476847, 0)
  point P0 (0, 0)
  constraints: 2 end point, 1 coincident, 1 horizontal
sketch "Эскиз29" plane through (0, 6, 0) normal (0, 1, 0) x (1, 0, 0)
  line L0 (294.632372, 46.383087) -> (294.632372, 42.383087)
  line L1 (294.632372, 42.383087) -> (296.632372, 42.383087)
  line L2 (296.632372, 42.383087) -> (296.632372, 46.383087)
  line L3 (296.632372, 46.383087) -> (294.632372, 46.383087)
  line L4 (316.632372, 46.383087) -> (316.632372, 42.383087)
  line L5 (316.632372, 42.383087) -> (318.632372, 42.383087)
  line L6 (318.632372, 42.383087) -> (318.632372, 46.383087)
  line L7 (318.632372, 46.383087) -> (316.632372, 46.383087)
  line L8 (249.114929, 89.848298) -> (249.114929, 89.848298)
  line L9 (249.114929, 109.848298) -> (249.114929, 109.848298)
  point P0 (0, 0)
  dimension "d183" = 2
  dimension "d184" = 4
  dimension "d185" = 20
  constraints: 20 end point, 4 parallel, 3 equal length, 2 perpendicular, 1 collinear, 1 point on line, 1 vertical
  measures "d183" distance of L2.end L0.start
  measures "d184" distance of L0.start L0.end
  measures "d185" distance between parallel lines of L4 L2
extrude "Выдавливание34" cut sketch "Эскиз29" against normal blind 6
extrude "Выдавливание35" cut sketch "Эскиз25" against normal blind 6 contours A7 | A8 | A9 | A10
extrude "Выдавливание39" cut sketch "Эскиз19" against normal blind 6 contours A30
sketch "Эскиз31" plane through (0, 6, 0) normal (0, 1, 0) x (1, 0, 0)
  point P0 (0, 0)
extrude "Выдавливание41" cut sketch "Эскиз25" against normal blind 6 contours L5 L4 L3 L2 | L9 L8 L7 L6 | L10 L11 L12 L13 | L14 L15 L16 L17
extrude "Выдавливание42" cut sketch "Эскиз19" against normal blind 6 contours A33 | A34 | A35 | A36
sketch "Эскиз32" plane through (0, 6, 0) normal (0, 1, 0) x (1, 0, 0)
  point P0 (0, 0)
sketch "Эскиз33" plane through (0, 0, 0) normal (0, -1, 0) x (1, 0, 0)
  line L0 (222.921453, 19.972322) -> (222.921453, 59.916966)
  line L1 (222.921453, 19.972322) -> (312.921453, 19.972322)
  line L2 (-118.106808, 0) -> (708.640848, 0)
  line L3 (312.921453, 19.972322) -> (312.921453, 0)
  point P0 (0, 0)
  dimension "d222" = 90
  constraints: 4 end point, 1 horizontal, 1 point on line, 1 vertical
  measures "d222" distance of L0.start L1.end
sketch "Эскиз35" plane through (0, 6, 0) normal (0, 1, 0) x (1, 0, 0)
  line L0 (337.023489, -2) -> (337.023489, 2)
  line L1 (338.102036, -47.843891) -> (338.102036, 47.843891)
  point P0 (0, 0)
  constraints: 2 end point, 1 vertical, 2 other
extrude "Выдавливание45" cut sketch "Эскиз27" against normal blind 6 contours A2 | A3 | A4 | A5
extrude "Выдавливание47" cut sketch "Эскиз20" against normal blind 6 contours A5 L13 | L13 A5
extrude "Выдавливание48" cut sketch "Эскиз25" against normal blind 6 contours L21 L20 L19 L18 | L25 L24 L23 L22
extrude "Выдавливание49" cut sketch "Эскиз25" against normal blind 6 contours A11 | A12
extrude "Выдавливание50" cut sketch "Эскиз25" against normal blind 6 contours A13 | A14
extrude "Выдавливание51" add sketch "Эскиз20" against normal blind 6 contours S1 A4 A9 A10 L6
